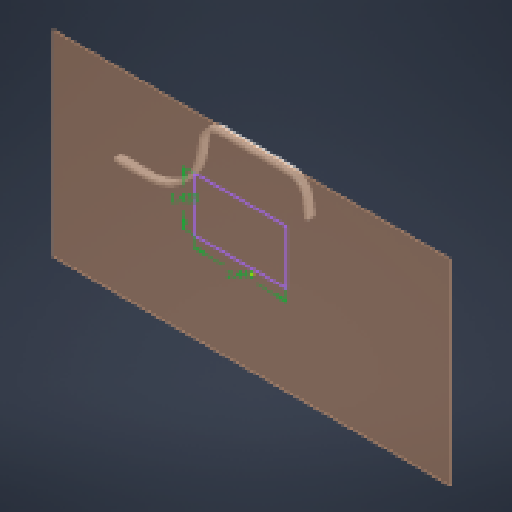
# Autodesk Inventor part: MISLCaseV2
Saved by Autodesk Inventor 2026.1 (Build 301233020, 233B)
## iProperties
Created: 2026-09-27
Part Number: MISLCaseV2
Material: Generic
Document SubType Name: Modeling
Density: 1 g/cm^3
Appearance: Default
Autodesk Inventor part; units mm, degrees
ref_plane "YZ Plane" through (0, 0, 0) normal (1, 0, 0) x (0, 1, 0)
ref_plane "XZ Plane" through (0, 0, 0) normal (0, 1, 0) x (-1, 0, 0)
ref_plane "XY Plane" through (0, 0, 0) normal (0, 0, 1) x (1, 0, 0)
ref_plane "Work Plane1" through (0, 0, 0) normal (0, 0, 1) x (1, 0, 0)
ref_plane "Work Plane2" through (0, 0, 0) normal (0, 0, 1) x (1, 0, 0)
sketch "Sketch2" plane through (0, 0, 0) normal (0, 0, 1) x (1, 0, 0)
  line L0 (30.0744, 9.362) -> (30.0744, 6.151) projected
  line L1 (30.0744, 6.151) -> (35.4879, 6.151) projected
  line L2 (35.4879, 6.151) -> (35.4879, 3.7325) projected
  line L3 (35.4879, 3.7325) -> (26.9046, 3.7325) projected
  line L4 (26.9046, 3.7325) -> (26.9046, 16.4325) projected
  line L5 (26.9046, 16.4325) -> (35.4879, 16.4325) projected
  line L6 (35.4879, 16.4325) -> (35.4879, 14.0139) projected
  line L7 (35.4879, 14.0139) -> (30.0744, 14.0139) projected
  line L8 (30.0744, 14.0139) -> (30.0744, 11.7806) projected
  line L9 (30.0744, 11.7806) -> (35.0659, 11.7806) projected
  line L10 (35.0659, 11.7806) -> (35.0659, 9.362) projected
  line L11 (35.0659, 9.362) -> (30.0744, 9.362) projected
  line L12 (-20.6844, 16.4325) -> (-15.5797, 16.4325) projected
  spline S0 degree 2 poles (-15.5797, 16.4325) (-14.5196, 16.4325) (-12.9553, 16.1649) (-12.2863, 15.7532) knots 0 0 0 1 2 2 2 projected
  spline S1 degree 2 poles (-12.2863, 15.7532) (-11.6071, 15.321) (-10.8043, 13.9727) (-10.8043, 12.9436) knots 0 0 0 1 2 2 2 projected
  spline S2 degree 2 poles (-10.8043, 12.9436) (-10.8043, 11.4924) (-12.1217, 9.6708) (-13.2229, 9.1356) knots 0 0 0 1 2 2 2 projected
  line L13 (-13.2229, 9.1356) -> (-8.9518, 3.7325) projected
  line L14 (-8.9518, 3.7325) -> (-12.8318, 3.7325) projected
  line L15 (-12.8318, 3.7325) -> (-16.3619, 8.3946) projected
  line L16 (-16.3619, 8.3946) -> (-17.5145, 8.3946) projected
  line L17 (-17.5145, 8.3946) -> (-17.5145, 3.7325) projected
  line L18 (-17.5145, 3.7325) -> (-20.6844, 3.7325) projected
  line L19 (-20.6844, 3.7325) -> (-20.6844, 16.4325) projected
  line L20 (-30.832, 3.7325) -> (-30.832, 16.4325) projected
  line L21 (-30.832, 16.4325) -> (-22.3311, 16.4325) projected
  line L22 (-22.3311, 16.4325) -> (-22.3311, 14.0139) projected
  line L23 (-22.3311, 14.0139) -> (-27.6622, 14.0139) projected
  line L24 (-27.6622, 14.0139) -> (-27.6622, 11.6159) projected
  line L25 (-27.6622, 11.6159) -> (-22.753, 11.6159) projected
  line L26 (-22.753, 11.6159) -> (-22.753, 9.1974) projected
  line L27 (-22.753, 9.1974) -> (-27.6622, 9.1974) projected
  line L28 (-27.6622, 9.1974) -> (-27.6622, 3.7325) projected
  line L29 (-27.6622, 3.7325) -> (-30.832, 3.7325) projected
  line L30 (-1.6858, 16.4325) -> (-1.6858, 14.2197) projected
  line L31 (-1.6858, 14.2197) -> (-3.5075, 14.2197) projected
  line L32 (-3.5075, 14.2197) -> (-3.5075, 5.9452) projected
  line L33 (-3.5075, 5.9452) -> (-1.6858, 5.9452) projected
  line L34 (-1.6858, 5.9452) -> (-1.6858, 3.7325) projected
  line L35 (-1.6858, 3.7325) -> (-8.5196, 3.7325) projected
  line L36 (-8.5196, 3.7325) -> (-8.5196, 5.9452) projected
  line L37 (-8.5196, 5.9452) -> (-6.6979, 5.9452) projected
  line L38 (-6.6979, 5.9452) -> (-6.6979, 14.2197) projected
  line L39 (-6.6979, 14.2197) -> (-8.5196, 14.2197) projected
  line L40 (-8.5196, 14.2197) -> (-8.5196, 16.4325) projected
  line L41 (-8.5196, 16.4325) -> (-1.6858, 16.4325) projected
  line L42 (8.4001, 9.1562) -> (8.4001, 16.4325) projected
  line L43 (8.4001, 16.4325) -> (11.3126, 16.4325) projected
  line L44 (11.3126, 16.4325) -> (11.3126, 3.7325) projected
  line L45 (11.3126, 3.7325) -> (8.2457, 3.7325) projected
  line L46 (8.2457, 3.7325) -> (3.3468, 12.5834) projected
  line L47 (3.3468, 12.5834) -> (3.3468, 3.7325) projected
  line L48 (3.3468, 3.7325) -> (0.4343, 3.7325) projected
  line L49 (0.4343, 3.7325) -> (0.4343, 16.4325) projected
  line L50 (0.4343, 16.4325) -> (4.3451, 16.4325) projected
  line L51 (4.3451, 16.4325) -> (8.4001, 9.1562) projected
  spline S3 degree 2 poles (17.5391, 13.2729) (17.0348, 12.7583) (16.4482, 11.1837) (16.4482, 10.1442) knots 0 0 0 1 2 2 2 projected
  spline S4 degree 2 poles (16.4482, 10.1442) (16.4482, 7.9212) (18.6815, 5.8011) (20.606, 5.8011) knots 0 0 0 1 2 2 2 projected
  spline S5 degree 2 poles (20.606, 5.8011) (20.781, 5.8011) (21.2338, 5.8217) (21.4088, 5.832) knots 0 0 0 1 2 2 2 projected
  line L52 (21.4088, 5.832) -> (21.4088, 8.3329) projected
  line L53 (21.4088, 8.3329) -> (18.9491, 8.3329) projected
  line L54 (18.9491, 8.3329) -> (18.9491, 10.7103) projected
  line L55 (18.9491, 10.7103) -> (24.4963, 10.7103) projected
  line L56 (24.4963, 10.7103) -> (24.4963, 4.4529) projected
  spline S6 degree 2 poles (24.4963, 4.4529) (23.6627, 4.1133) (20.9971, 3.4649) (19.7004, 3.4649) knots 0 0 0 1 2 2 2 projected
  spline S7 degree 2 poles (19.7004, 3.4649) (16.7055, 3.4649) (13.1548, 6.9229) (13.1548, 10.0928) knots 0 0 0 1 2 2 2 projected
  spline S8 degree 2 poles (13.1548, 10.0928) (13.1548, 13.0774) (16.7055, 16.6795) (19.793, 16.6795) knots 0 0 0 1 2 2 2 projected
  spline S9 degree 2 poles (19.793, 16.6795) (21.3882, 16.6795) (23.3848, 16.0722) (24.4449, 15.5577) knots 0 0 0 1 2 2 2 projected
  line L57 (24.4449, 15.5577) -> (24.4449, 12.5731) projected
  line L58 (24.4449, 12.5731) -> (24.1567, 12.5731) projected
  spline S10 degree 2 poles (24.1567, 12.5731) (23.9303, 12.748) (23.0658, 13.417) (22.6541, 13.6434) knots 0 0 0 1 2 2 2 projected
  spline S11 degree 2 poles (22.6541, 13.6434) (22.1807, 13.9213) (20.9251, 14.3124) (20.2253, 14.3124) knots 0 0 0 1 2 2 2 projected
  spline S12 degree 2 poles (20.2253, 14.3124) (19.4122, 14.3124) (18.064, 13.7978) (17.5391, 13.2729) knots 0 0 0 1 2 2 2 projected
  line L59 (-121.793, -38.1) -> (-93.218, -38.1) projected
  line L60 (-93.218, 0) -> (-93.218, -38.1) projected
  line L61 (-93.218, 0) -> (93.218, 0) projected
  line L62 (93.218, 0) -> (93.218, -38.1) projected
  line L63 (93.218, -38.1) -> (121.4251, -38.1) projected
  line L64 (121.4251, -38.1) -> (121.4251, -50.8) projected
  line L65 (121.793, -50.8) -> (121.4251, -50.8) projected
  line L66 (121.793, -50.8) -> (121.793, 12.7) projected
  arc A0 (121.793, 12.7) -> (115.443, 19.05) centre (115.443, 12.7) ccw projected
  line L67 (115.443, 19.05) -> (72.4101, 19.05) projected
  arc A1 (34.8023, 51.0455) -> (72.4101, 19.05) centre (72.4101, 57.15) ccw projected
  line L68 (33.1349, 61.3179) -> (34.8023, 51.0455) projected
  arc A2 (33.1349, 61.3179) -> (23.1062, 69.85) centre (23.1062, 59.69) ccw projected
  line L69 (-23.1062, 69.85) -> (23.1062, 69.85) projected
  arc A3 (-23.1062, 69.85) -> (-33.1349, 61.3179) centre (-23.1062, 59.69) ccw projected
  line L70 (-34.8023, 51.0455) -> (-33.1349, 61.3179) projected
  arc A4 (-72.4101, 19.05) -> (-34.8023, 51.0455) centre (-72.4101, 57.15) ccw projected
  line L71 (-115.443, 19.05) -> (-72.4101, 19.05) projected
  arc A5 (-115.443, 19.05) -> (-121.793, 12.7) centre (-115.443, 12.7) ccw projected
  line L72 (-121.793, 12.7) -> (-121.793, -38.1) projected
  circle A6 centre (0, 50.8) radius 3.9687 projected
  line L73 (-35.2959, 51.1256) -> (-33.6285, 61.398)
  arc A7 (-23.1062, 70.35) -> (-33.6285, 61.398) centre (-23.1062, 59.69) ccw
  line L74 (-23.1062, 70.35) -> (23.1062, 70.35)
  arc A8 (33.6285, 61.398) -> (23.1062, 70.35) centre (23.1062, 59.69) ccw
  line L75 (33.6285, 61.398) -> (35.2959, 51.1256)
  arc A9 (35.2959, 51.1256) -> (35.4879, 50.0429) centre (72.4101, 57.15) ccw
  line L76 (93.218, -38.6) -> (92.718, -38.6)
  line L77 (92.718, -38.6) -> (92.718, -38.1)
  line L78 (-92.718, -38.1) -> (-92.718, -38.6)
  line L79 (-93.218, 19.55) -> (-72.4101, 19.55)
  arc A10 (-72.4101, 19.55) -> (-35.2959, 51.1256) centre (-72.4101, 57.15) ccw
  line L80 (-92.718, -38.6) -> (-93.218, -38.6)
  line L81 (-121.793, -38.6) -> (-122.293, -38.6)
  line L82 (-122.293, -38.6) -> (-122.293, -38.1)
  line L83 (-122.293, -0.5) -> (-122.293, 0)
  line L84 (92.718, 19.55) -> (93.218, 19.55)
  arc A11 (37.27, 51.4461) -> (37.4518, 50.421) centre (72.4101, 57.15) ccw
  line L85 (37.27, 51.4461) -> (35.6026, 61.7184)
  arc A12 (35.6026, 61.7184) -> (23.1062, 72.35) centre (23.1062, 59.69) ccw
  line L86 (23.1062, 72.35) -> (-23.1062, 72.35)
  arc A13 (-23.1062, 72.35) -> (-35.6026, 61.7184) centre (-23.1062, 59.69) ccw
  line L87 (-35.6026, 61.7184) -> (-37.27, 51.4461)
  arc A14 (-72.4101, 21.55) -> (-37.27, 51.4461) centre (-72.4101, 57.15) ccw
  line L88 (-72.4101, 21.55) -> (-93.218, 21.55)
  line L89 (-93.218, 21.55) -> (-93.218, 19.55)
  line L90 (37.4518, 50.421) -> (35.4879, 50.0429)
  point P0 (0, 0)
  point P1 (-81.8285, 19.05)
  point P2 (-81.8285, 19.55)
  point P3 (-81.8285, 19.55)
  dimension "d0" = 0.5
  dimension "d1" = 2
  constraints: 36 end point, 16 point on circle, 13 point on line, 8 centre point, 3 coincident, 1 vertical, 11 other
  measures "d0" radial gap between concentric circles of A4 A10
  measures "d1" radial gap between concentric circles of A10 A14
extrude "Frame offset outline holder" add sketch "Sketch2" against normal blind 5.08 contours A10 L79 L89 L88 A14 L87 A13 L86 A12 L85 A11 L90 A9 L75 A8 L74 A7 L73
sketch "Sketch3" plane through (0, 0, 0) normal (0, 0, 1) x (1, 0, 0)
  line L0 (-76.4813, 63.2926) -> (-76.4813, 26.7926)
  line L1 (-76.4813, 26.7926) -> (-14.4813, 26.7926)
  line L2 (-14.4813, 26.7926) -> (-14.4813, 63.2926)
  line L3 (-14.4813, 63.2926) -> (-76.4813, 63.2926)
  circle A0 centre (0, 50.8) radius 6.35 projected
  circle A1 centre (0, 50.8) radius 7.62
  circle A2 centre (0, 50.8) radius 8.89
  line L4 (35.4879, 50.0429) -> (37.4518, 50.421) projected
  line L5 (-76.4813, 26.7926) -> (-76.4813, 24.2526)
  line L6 (-93.218, 21.55) -> (-93.218, 19.55) projected
  line L7 (-93.218, 19.55) -> (-72.4101, 19.55) projected
  arc A3 (-72.4101, 19.55) -> (-35.2959, 51.1256) centre (-72.4101, 57.15) ccw projected
  line L8 (-35.2959, 51.1256) -> (-33.6285, 61.398) projected
  arc A4 (-23.1062, 70.35) -> (-33.6285, 61.398) centre (-23.1062, 59.69) ccw projected
  line L9 (-23.1062, 70.35) -> (23.1062, 70.35) projected
  arc A5 (33.6285, 61.398) -> (23.1062, 70.35) centre (23.1062, 59.69) ccw projected
  line L10 (33.6285, 61.398) -> (35.2959, 51.1256) projected
  arc A6 (35.2959, 51.1256) -> (35.4879, 50.0429) centre (72.4101, 57.15) ccw projected
  line L11 (35.4879, 50.0429) -> (37.4518, 50.421) projected
  arc A7 (37.27, 51.4461) -> (37.4518, 50.421) centre (72.4101, 57.15) ccw projected
  line L12 (37.27, 51.4461) -> (35.6026, 61.7184) projected
  arc A8 (35.6026, 61.7184) -> (23.1062, 72.35) centre (23.1062, 59.69) ccw projected
  line L13 (23.1062, 72.35) -> (-23.1062, 72.35) projected
  arc A9 (-23.1062, 72.35) -> (-35.6026, 61.7184) centre (-23.1062, 59.69) ccw projected
  line L14 (-35.6026, 61.7184) -> (-37.27, 51.4461) projected
  arc A10 (-72.4101, 21.55) -> (-37.27, 51.4461) centre (-72.4101, 57.15) ccw projected
  line L15 (-72.4101, 21.55) -> (-93.218, 21.55) projected
  line L16 (-14.4813, 63.2926) -> (-14.4813, 53.1326)
  line L17 (37.4518, 50.421) -> (6.1698, 44.3996)
  line L18 (-14.4813, 26.7926) -> (-14.4813, 36.9526)
  line L19 (-14.4813, 36.9526) -> (-11.9413, 36.9526)
  line L20 (-11.9413, 36.9526) -> (-11.9413, 53.1326)
  line L21 (-11.9413, 53.1326) -> (-14.4813, 53.1326)
  line L22 (-14.4813, 26.7926) -> (-14.4813, 24.2526)
  line L23 (-14.4813, 24.2526) -> (0, 41.91)
  line L24 (-14.4813, 24.2526) -> (-76.4813, 24.2526)
  line L25 (-76.4813, 24.2526) -> (-79.0213, 24.2526)
  line L26 (-79.0213, 24.2526) -> (-79.0213, 63.2926)
  line L27 (-79.0213, 63.2926) -> (-79.0213, 65.8326)
  line L28 (-79.0213, 65.8326) -> (-34.1761, 65.8326)
  line L29 (-79.0213, 24.2526) -> (-79.0213, 21.55)
  circle A11 centre (0, 50.8) radius 4.826 projected
  circle A12 centre (0, 50.8) radius 6.35 projected
  circle A13 centre (0, 50.8) radius 9.525 projected
  point P0 (0, 0)
  point P1 (-54.2023, 24.2526)
  dimension "d4" = 36.5
  dimension "d5" = 62
  dimension "d6" = 15.24
  dimension "d7" = 17.78
  dimension "d8" = 2.54
  dimension "d9" = 10.16
  dimension "d11" = 10.16
  dimension "d12" = 2.54
  dimension "d13" = 2.54
  dimension "d14" = 2.54
  dimension "d15" = 2.54
  constraints: 38 end point, 7 perpendicular, 6 point on line, 3 point on circle, 3 vertical, 2 centre point, 2 coincident, 2 parallel
  measures "d4" distance of L0.start L0.end
  measures "d5" distance of L1.end L0.end
  measures "d6" diameter of A1
  measures "d7" diameter of A2
  measures "d8" distance of L0.end L5.end
  measures "d9" distance of L2.end L16.end
  measures "d11" distance of L1.end L18.end
  measures "d12" distance of L18.end L19.end
  measures "d13" distance of L1.end L22.end
  measures "d14" distance of L5.end L25.end
  measures "d15" distance of L26.end L27.end
extrude "backplate 1" add sketch "Sketch3" along normal blind 2 contours L3 A9 L14 A10 L1 L0 | L0 L5 L25 L26 L27 L28 A9 L3 | L1 A10 L24 L5 | A9 L13 A8 L12 A7 L4 A6 L10 A5 L9 A4 L3 | L3 A4 L8 A3 L1 A10 L14 A9 | L1 A3 L24 A10 | L24 A10 L15 L29 L25 | A4 L9 A5 L10 A6 L17 A13 L23 L22 L2 L19 L20 L21 L3 | L3 L2 L1 A3 L8 A4 | L1 L22 L24 A3 | L24 A3 L7 L6 L15 A10 | L21 L20 L19 L2 | A13 L17 A2 L23 | A2 | A0 | A1 picked at (-0.8973, 41.7936)
sketch "Sketch4" plane through (0, 0, 2) normal (0, 0, 1) x (1, 0, 0)
  circle A0 centre (0, 50.8) radius 8.89 projected
  circle A1 centre (0, 50.8) radius 7.62 projected
  point P0 (0, 0)
extrude "Bolt holder" add sketch "Sketch4" along normal blind 4
fillet "Fillet1" radius 0.7 3 edges at (-7.62, 50.8, 2) (-6.2862, 57.0862, 2) (8.1817, 47.3228, 2)
sketch "Sketch5" plane through (0, 0, 2) normal (0, 0, 1) x (1, 0, 0)
  line L0 (-14.4813, 26.7926) -> (-14.4813, 63.2926) projected
  line L1 (-11.9413, 53.1326) -> (-14.4813, 53.1326) projected
  line L2 (-11.9413, 36.9526) -> (-11.9413, 53.1326) projected
  line L3 (-14.4813, 36.9526) -> (-11.9413, 36.9526) projected
  line L4 (-76.4813, 26.7926) -> (-14.4813, 26.7926) projected
  line L5 (-76.4813, 63.2926) -> (-76.4813, 26.7926) projected
  line L6 (-14.4813, 24.2526) -> (-76.4813, 24.2526) projected
  line L7 (-14.4813, 26.7926) -> (-14.4813, 24.2526) projected
  line L8 (-14.4813, 63.2926) -> (-76.4813, 63.2926) projected
  line L9 (-34.1761, 65.8326) -> (-79.0213, 65.8326) projected
  line L10 (-79.0213, 65.8326) -> (-79.0213, 21.55) projected
  line L11 (-76.4813, 24.2526) -> (-79.0213, 24.2526) projected
  line L12 (-76.4813, 26.7926) -> (-76.4813, 24.2526) projected
  line L13 (-76.4813, 26.7926) -> (-66.3213, 26.7926)
  line L14 (-66.3213, 26.7926) -> (-66.3213, 24.2526)
  line L15 (-14.4813, 26.7926) -> (-24.6413, 26.7926)
  line L16 (-24.6413, 26.7926) -> (-24.6413, 24.2526)
  line L17 (-34.1761, 65.8326) -> (-14.4813, 65.8326)
  line L18 (-14.4813, 65.8326) -> (-14.4813, 63.2926)
  line L19 (-14.4813, 65.8326) -> (-24.6413, 65.8326)
  line L20 (-24.6413, 65.8326) -> (-24.6413, 63.2926)
  line L21 (-76.4813, 65.8326) -> (-66.3213, 65.8326)
  line L22 (-66.3213, 65.8326) -> (-66.3213, 63.2926)
  line L23 (-76.4813, 63.2926) -> (-76.4813, 58.2126)
  line L24 (-76.4813, 58.2126) -> (-79.0213, 58.2126)
  line L25 (-76.4813, 26.7926) -> (-76.4813, 31.8726)
  line L26 (-76.4813, 31.8726) -> (-79.0213, 31.8726)
  point P0 (0, 0)
  dimension "d21" = 10.16
  dimension "d22" = 10.16
  dimension "d23" = 10.16
  dimension "d24" = 10.16
  dimension "d25" = 5.08
  dimension "d26" = 5.08
  constraints: 28 end point, 15 point on line, 5 perpendicular, 1 horizontal
  measures "d21" distance of L4.start L13.end
  measures "d22" distance of L0.start L15.end
  measures "d23" distance of L17.end L19.end
  measures "d24" distance of L21.start L21.end
  measures "d25" distance of L5.start L23.end
  measures "d26" distance of L4.start L25.end
extrude "Extrusion4" add sketch "Sketch5" along normal blind 19.05 contours L0 L1 L2 L3 | L16 L6 L14 L4 | L8 L22 L9 L17 L20 | L26 L10 L24 L5
sketch "Sketch6" plane through (0, 0, -5.08) normal (0, 0, -1) x (-1, 0, 0)
  circle A0 centre (51.2954, 76.7254) radius 2.5
  circle A1 centre (51.2954, 76.7254) radius 4.5
  circle A2 centre (51.2954, 76.7254) radius 1.25
  point P0 (0, 0)
  dimension "d31" = 5
  dimension "d32" = 2
  dimension "d33" = 2.5
  constraints: 3 centre point, 1 coincident
  measures "d31" diameter of A0
  measures "d32" radial gap between concentric circles of A0 A1
  measures "d33" diameter of A2
extrude "aperture plate" add sketch "Sketch6" against normal blind 2 contours A0 | A1
sketch "Sketch7" plane through (-51.2954, 76.7254, -3.08) normal (0, 0, 1) x (1, 0, 0)
  circle A0 centre (0, 0) radius 2.5 projected
  circle A1 centre (0, 0) radius 4.5 projected
  point P0 (51.2954, -76.7254)
extrude "emitter tube" add sketch "Sketch7" along normal blind 11
fillet "Fillet2" radius 2 4 edges at (-75.7157, 21.55, 0) (-36.4363, 56.5823, 0) (-35.0676, 63.8373, 0) (-49.3417, 30.0353, 0)
fillet "Fillet3" radius 1 1 edges at (-53.7954, 76.7254, -3.08)
sketch "Sketch8" plane through (0, 0, 0) normal (0, 0, -1) x (-1, 0, 0)
  circle A0 centre (51.2954, 76.7254) radius 4.5 projected
  line L0 (46.7954, 76.7254) -> (46.7954, 63.2926)
  line L1 (24.6413, 63.2926) -> (66.3213, 63.2926) projected
  line L2 (55.7954, 76.7254) -> (55.7954, 63.2926)
  point P0 (0, 0)
  constraints: 4 end point, 2 point on circle, 2 vertical, 1 point on line
extrude "Extrusion7" add sketch "Sketch8" along normal blind 5.08 contours L2 L1 L0 A0
chamfer "Chamfer1" distance 2.54 angle 45 2 edges at (-51.2954, 63.2926, 0) (-51.2954, 63.2926, -5.08)
chamfer "Chamfer2" distance 2.54 angle 45 1 edges at (-51.2954, 65.8326, 0)
sketch "Sketch9" plane through (0, 0, 0) normal (0, 0, -1) x (-1, 0, 0)
  line L0 (55.7954, 65.8326) -> (46.7954, 65.8326) projected
  line L1 (24.6413, 65.8326) -> (66.3213, 65.8326) projected
  line L2 (51.3037, 65.8326) -> (49.3037, 65.8326)
  line L3 (51.3037, 65.8326) -> (53.3037, 65.8326)
  line L4 (49.3037, 65.8326) -> (49.3037, 27.4876)
  arc A0 (35.2959, 51.1256) -> (54.2023, 24.2526) centre (72.4101, 57.15) ccw projected
  line L5 (53.3037, 65.8326) -> (53.3037, 26.7926)
  line L6 (66.3213, 26.7926) -> (24.6413, 26.7926) projected
  line L7 (49.3037, 27.4876) -> (53.3037, 27.4876)
  line L8 (49.3037, 27.4876) -> (53.3037, 26.7926)
  point P0 (0, 0)
  dimension "d48" = 2
  dimension "d49" = 2
  constraints: 12 end point, 5 point on line, 2 vertical, 1 perpendicular, 1 point on circle
  measures "d48" distance of L2.start L2.end
  measures "d49" distance of L2.start L3.end
extrude "Extrusion9" add sketch "Sketch9" along normal blind 2 contours L5 L7 L4 L0 | L5 L8 L7
body "Solid1"
